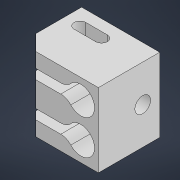
# Autodesk Inventor part: Component94
Saved by Autodesk Inventor 2022 (Build 260153000, 153)
## iProperties
Created: 2021-10-06
Part Number: Component94
Material: Generic
Document SubType Name: Modeling
Designer: Administrator
Density: 1 g/cm^3
Appearance: Default
Mass: 1.15028 g
Surface Area: 12.4989 cm^2
Volume: 1.15028 cm^3
Title: Component94
Author: Administrator
Autodesk Inventor part; units mm, degrees
ref_plane "YZ Plane" through (0, 0, 0) normal (1, 0, 0) x (0, 1, 0)
ref_plane "Work Plane1" through (0, 33.012, 0) normal (0, 1, 0) x (-1, 0, 0)
ref_plane "Work Plane2" through (0, 0, 19.2509) normal (0, 0, 1) x (1, 0, 0)
sketch "Sketch1" plane through (0, 33.012, 0) normal (0, 1, 0) x (-1, 0, 0)
  line L0 (12.3254, 14.5509) -> (12.3254, 30.2509)
  line L1 (20.3254, 14.5509) -> (12.3254, 14.5509)
  line L2 (12.3254, 30.2509) -> (20.3254, 30.2509)
  line L3 (20.3254, 30.2509) -> (20.3254, 14.5509)
  constraints: 8 end point, 2 horizontal, 2 vertical
extrude "Extrusion12" add sketch "Sketch1" along normal blind 17
sketch "Sketch2" plane through (-20.3254, 33.012, 30.2509) normal (0, 0, 1) x (1, 0, 0)
  arc A0 (0.2308, 10.75) -> (0.2308, 13.25) centre (3.5, 12) ccw
  line L0 (-0.0992, 10.75) -> (-0.0992, 13.25)
  line L1 (0.2308, 10.75) -> (-0.0992, 10.75)
  line L2 (0.2308, 13.25) -> (-0.0992, 13.25)
  circle A1 centre (3.5, 12) radius 1.5
  dimension "d52" = 2.5
  dimension "d66" = 3
  dimension "d67" = 2
  constraints: 6 end point, 2 centre point, 2 horizontal, 2 point on circle, 1 coincident, 1 parallel, 1 vertical, 1 other
  measures "d52" distance of L0.start L0.end
  measures "d66" diameter of A1
  measures "d67" radial gap between concentric circles of A0 A1
extrude "Extrusion11" cut sketch "Sketch2" against normal blind 7 draft 0 contours L1 L0 L2 A0 | A1
sketch "Sketch3" plane through (-20.3254, 33.012, 14.5509) normal (-1, 0, 0) x (0, 0, 1)
  line L0 (6.75, 5.0877) -> (6.75, 0)
  line L1 (1.25, 0) -> (1.25, 5.0877)
  line L2 (4, 6.6754) -> (6.75, 5.0877)
  line L3 (1.25, 5.0877) -> (4, 6.6754)
  line L4 (6.75, 0) -> (1.25, 0)
  constraints: 10 end point, 2 equal length, 2 vertical, 1 horizontal
extrude "Extrusion10" cut sketch "Sketch3" against normal blind 2.5
sketch "Sketch4" plane through (0, 33.012, 0) normal (0, 1, 0) x (-1, 0, 0)
  line L0 (12.3254, 30.2509) -> (31.3754, 30.2509)
  line L1 (20.3254, 14.5509) -> (20.3254, 22.5509)
  line L2 (12.3254, 22.5509) -> (12.3254, 30.2509)
  line L3 (20.3254, 14.5509) -> (31.3754, 14.5509)
  line L4 (20.3254, 22.5509) -> (12.3254, 22.5509)
  line L5 (31.3754, 30.2509) -> (31.3754, 14.5509)
  constraints: 12 end point, 3 horizontal, 3 vertical, 1 perpendicular
extrude "Extrusion9" cut sketch "Sketch4" along normal blind 7 draft 0
sketch "Sketch12" plane through (-20.3254, 50.012, 30.2509) normal (0, 0, 1) x (1, 0, 0)
  line L0 (0, -17) -> (0, 0) projected
  line L1 (0, 0) -> (-12, 0)
  line L2 (-12, 0) -> (-12, -10)
  line L3 (-12, -10) -> (0, -10)
  line L4 (0, -10) -> (0, 0)
  line L5 (0, -6.25) -> (0, -3.75) projected
  line L6 (0, -3.75) -> (-13.6518, -3.75)
  line L7 (-13.6518, -3.75) -> (-13.6518, -6.25)
  line L8 (-13.6518, -6.25) -> (0, -6.25)
  line L9 (0, -6.25) -> (0, -3.75)
  line L10 (0, -10) -> (8, -10) projected
  line L11 (8, -10) -> (8, 0) projected
  point P0 (20.3254, -50.012)
  point P1 (-12, -6.25)
  point P2 (-12, -3.75)
  dimension "d44" = 20
  constraints: 16 end point, 4 parallel, 2 horizontal, 2 perpendicular, 1 collinear
  measures "d44" distance between parallel lines of L11 L2
extrude "Extrusion15" add sketch "Sketch12" against normal up to surface (15.7 mm away) contours L3 L2 L8 L0 | L8 L2 L6 L0 | L6 L2 L1 L0
extrude "Extrusion16" cut sketch "Sketch12" against normal up to surface (7 mm away) contours L8 L2 L6 L0
sketch "Sketch6" plane through (0, 40.012, 0) normal (0, -1, 0) x (1, 0, 0)
  line L0 (-22.8754, 17.4009) -> (-28.3754, 17.4009)
  arc A0 (-28.3754, 20.4009) -> (-28.3754, 17.4009) centre (-28.3754, 18.9009) ccw
  line L1 (-28.3754, 20.4009) -> (-22.8754, 20.4009)
  arc A1 (-22.8754, 17.4009) -> (-22.8754, 20.4009) centre (-22.8754, 18.9009) ccw
  constraints: 4 end point, 4 point on circle, 2 centre point, 2 horizontal, 1 equal radius, 1 parallel
extrude "Extrusion7" cut sketch "Sketch6" against normal blind 10 draft 0
sketch "Sketch7" plane through (-12.3254, 33.012, 14.5509) normal (0, 0, -1) x (-1, 0, 0)
  point P0 (4.5, 12)
hole "Hole6" at (-16.8254, 45.012, 14.5509) direction (0, 0, 1) diameter 2.5 end through all
sketch "Sketch9" plane through (-17.8254, 33.012, 14.5509) normal (-1, 0, 0) x (0, 0, 1)
  point P0 (4, 3.5)
hole "Hole4" at (-17.8254, 36.512, 18.5509) direction (1, 0, 0) diameter 3 depth 5.5 tip angle 118
fillet "Fillet8" radius 2.5 1 edges at (-20.3254, 33.012, 21.9259)
fillet "Fillet7" radius 2.5 1 edges at (-20.3254, 33.012, 15.1759)
fillet "Fillet6" radius 3.5 1 edges at (-20.0946, 43.762, 26.7509)
fillet "Fillet5" radius 3.5 1 edges at (-20.0946, 46.262, 26.7509)
chamfer "Chamfer1" [suppressed]
chamfer "Chamfer2" distance 2 angle 45 2 edges at (-32.3254, 46.262, 26.7509) (-32.3254, 43.762, 26.7509)
sketch "Sketch14" plane through (-20.3254, 40.012, 22.5509) normal (0, 0, 1) x (1, 0, 0)
  arc A0 (0, -4.5) -> (2.5, -7) centre (2.5, -4.5) ccw projected
  line L0 (0, -1.9123) -> (0, -4.5) projected
  line L1 (0, -1.9123) -> (2.5, -1.9123) projected
  line L2 (2.5, -1.9123) -> (2.5, -7) projected
  line L3 (0, -1.9123) -> (2.5, -7)
  arc A1 (0, -4.5) -> (2.5, -7) centre (2.5, -4.5) ccw projected
  point P0 (20.3254, -40.012)
  point P1 (2.5, -7)
  constraints: 2 end point, 1 point on circle
extrude "Extrusion18" cut sketch "Sketch14" against normal blind 1.3875 contours L0 L3 A0
chamfer "Chamfer4" distance 4 angle 45 2 edges at (-32.3254, 49.137, 30.2509) (-32.3254, 40.887, 30.2509)
ref_plane "Work Plane3" through (-21.9672, 40.562, 30.2509) normal (0, 1, 0) x (1, 0, 0)
sketch "Sketch15" plane through (0, 33.012, 0) normal (0, -1, 0) x (1, 0, 0)
  line L0 (-25.3064, 10.3119) -> (-9.5646, 10.3119)
  line L1 (-9.5646, 10.3119) -> (-9.5646, 26.9005)
  line L2 (-9.5646, 26.9005) -> (-25.3064, 26.9005)
  line L3 (-25.3064, 26.9005) -> (-25.3064, 10.3119)
  point P0 (0, 0)
  constraints: 8 end point, 2 parallel, 1 horizontal, 1 perpendicular
extrude "Extrusion19" cut sketch "Sketch15" against normal up to surface (7 mm away)
mirror "Mirror1" about plane through (-21.9672, 40.562, 30.2509) normal (0, 1, 0)
sketch "Sketch16" plane through (-28.3254, 31.112, 30.2509) normal (0, -1, 0) x (1, 0, 0)
  line L0 (0, 0) -> (-4, -4) projected
  line L1 (-4, -4) -> (-4, -15.7) projected
  line L2 (16, -15.7) -> (-4, -15.7) projected
  line L3 (16, 0) -> (16, -15.7) projected
  line L4 (16, 0) -> (0, 0) projected
  arc A0 (5.45, -12.85) -> (5.45, -9.85) centre (5.45, -11.35) ccw projected
  line L5 (-0.05, -12.85) -> (5.45, -12.85) projected
  arc A1 (-0.05, -9.85) -> (-0.05, -12.85) centre (-0.05, -11.35) ccw projected
  line L6 (5.45, -9.85) -> (-0.05, -9.85) projected
  arc A2 (5.45, -14.55) -> (5.45, -8.15) centre (5.45, -11.35) ccw
  line L7 (5.45, -14.55) -> (-0.05, -14.55)
  arc A3 (-0.05, -8.15) -> (-0.05, -14.55) centre (-0.05, -11.35) ccw
  line L8 (-0.05, -8.15) -> (5.45, -8.15)
  point P0 (28.3254, -30.2509)
  dimension "d71" = 3.2
  constraints: 4 end point, 4 point on circle, 2 centre point, 3 other
  measures "d71" radius of A2
extrude "Extrusion20" cut sketch "Sketch16" against normal blind 15 contours L7 A3 L8 A2
sketch "Sketch18" plane through (-12.3254, 50.012, 30.2509) normal (1, 0, 0) x (0, 0, -1)
  circle A0 centre (11.35, -9.45) radius 2
  line L0 (15.7, -18.9) -> (15.7, 0) projected
  line L1 (15.7, -9.45) -> (7, -9.45) construction
  line L2 (7, -8.5) -> (7, -1.5) projected
  line L3 (7, -10.4) -> (7, -17.4) projected
  point P0 (30.2509, -50.012)
  point P1 (7, -2.625)
  point P2 (7, -7.375)
  point P3 (7, -16.275)
  point P4 (7, -11.525)
  dimension "d78" = 4
  constraints: 2 end point, 2 midpoint, 1 centre point, 1 coincident, 1 horizontal, 1 point on line
  measures "d78" diameter of A0
extrude "Extrusion22" cut sketch "Sketch18" against normal blind 5.7
sketch "Sketch19" plane through (-18.0254, 40.562, 18.9009) normal (1, 0, 0) x (0, 0, -1)
  circle A0 centre (0, 0) radius 2 projected
  circle A1 centre (0, 0) radius 1.5
  point P0 (18.9009, -40.562)
  dimension "d81" = 3
  constraints: 1 centre point, 1 coincident
  measures "d81" diameter of A1
extrude "Extrusion23" cut sketch "Sketch19" against normal blind 6.3625 contours A1
sketch "Sketch20" plane through (-32.3254, 41.762, 23.2509) normal (-1, 0, 0) x (0, 0, 1)
  circle A0 centre (-4.35, -1.2) radius 3.2
  circle A1 centre (-4.35, -1.2) radius 1.5 projected
  line L0 (-7.55, -10.65) -> (-7.55, 4.35) projected
  line L1 (-1.15, -10.65) -> (-1.15, 4.35) projected
  point P0 (-23.2509, -41.762)
  constraints: 1 centre point, 1 horizontal alignment, 1 tangent, 2 other
extrude "Extrusion24" cut sketch "Sketch20" against normal blind 6.3625 contours A0 | A1
body "Solid5"
